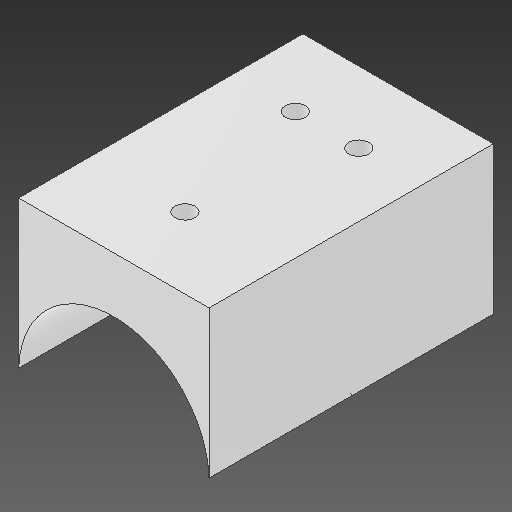
# Autodesk Inventor part: TopMotorMountSandwich3DPrint
Saved by Autodesk Inventor 2021 (Build 250183000, 183)
## iProperties
Created: 2021-02-22
Part Number: TopMotorMountSandwich3DPrint
Material: PC/ABS Plastic
Document SubType Name: Modeling
Designer: Esketitttttt
Density: 0.357273 g/cm^3
Appearance: Smooth - White
Mass: 0.946273 g
Surface Area: 18.8955 cm^2
Volume: 2.6486 cm^3
Author: Esketitttttt
Autodesk Inventor part; units mm, degrees
ref_plane "YZ Plane" through (0, 0, 0) normal (1, 0, 0) x (0, 1, 0)
ref_plane "XZ Plane" through (0, 0, 0) normal (0, 1, 0) x (-1, 0, 0)
ref_plane "XY Plane" through (0, 0, 0) normal (0, 0, 1) x (1, 0, 0)
sketch "Sketch1" plane through (0, 0, 0) normal (0, 0, 1) x (1, 0, 0)
  circle A0 centre (0, 0) radius 8.04
  line L0 (6, 4.8139) -> (6, -4.8139)
  arc A1 (6, 4.8139) -> (5.9407, 4.977) centre (5.746, 4.8139) ccw
  arc A2 (5.9407, 4.977) -> (-5.9407, 4.977) centre (0, 0) ccw
  arc A3 (-5.9407, 4.977) -> (-6, 4.8139) centre (-5.746, 4.8139) ccw
  line L1 (-6, -4.8139) -> (-6, 4.8139)
  arc A4 (-6, -4.8139) -> (-5.9407, -4.977) centre (-5.746, -4.8139) ccw
  arc A5 (-5.9407, -4.977) -> (5.9407, -4.977) centre (0, 0) ccw
  arc A6 (5.9407, -4.977) -> (6, -4.8139) centre (5.746, -4.8139) ccw
  line L2 (0, 8.04) -> (-12.7, 8.04)
  line L3 (0, 8.04) -> (12.7, 8.04) construction
  line L4 (-12.7, 8.04) -> (12.7, 8.04)
  line L5 (12.7, 8.04) -> (12.7, -8.04)
  line L6 (12.7, -8.04) -> (-12.7, -8.04)
  line L7 (-12.7, -8.04) -> (-12.7, 8.04)
  line L8 (0, -8.04) -> (0, 8.04)
  line L9 (0, 8.04) -> (0.254, 8.04)
  line L10 (0.254, 8.04) -> (0.254, -8.04)
  line L11 (0.254, -8.04) -> (0, -8.04)
  line L12 (0, -8.04) -> (0, 8.04)
  point P0 (0, -8.04)
  point P1 (0, -7.75)
  point P2 (0, 7.75)
  point P3 (0.254, 8.036)
  point P4 (0.254, -8.036)
  point P5 (0.254, -7.7458)
  point P6 (0.254, 7.7458)
  dimension "d0" = 12.7
  dimension "d2" = 25.4
  dimension "d7" = 0.254
  constraints: 26 end point, 12 point on circle, 6 centre point, 5 horizontal, 4 parallel, 2 perpendicular, 1 collinear, 1 midpoint, 1 point on line, 3 other
  measures "d0" distance of L2.start L2.end
  measures "d2" distance of L5.end L6.end
  measures "d7" distance of L10.end L11.end
extrude "Extrusion1" add sketch "Sketch1" along normal blind 12 contours L10 L4 L5 L6 A0
extrude "Extrusion2" add sketch "Sketch1" against normal blind 12 contours L10 L4 L5 L6 A0 | A0 L10 A5 A6 L0 A1 A2
sketch "Sketch2" plane through (12.7, -8.04, 12) normal (1, 0, 0) x (0, 0, -1)
  line L0 (12, 12.8539) -> (12, 3.2261) projected
  line L1 (24, 16.08) -> (24, 0) construction
  line L2 (24, 0) -> (0, 0) projected
  line L3 (24, 16.08) -> (12, 16.08)
  line L4 (12, 16.08) -> (12, 0)
  line L5 (12, 0) -> (24, 0)
  line L6 (24, 0) -> (24, 16.08) construction
  line L7 (24, 16.08) -> (0, 16.08) projected
  line L8 (12, 16.08) -> (24, 0) construction
  line L9 (12, 16.08) -> (16, 10.72) construction
  line L10 (16, 10.72) -> (20, 5.36) construction
  line L11 (12, 16.076) -> (0, 16.076) projected
  line L12 (12, 0) -> (0, 16.076)
  line L13 (24, 16.08) -> (18, 16.08)
  line L14 (18, 16.08) -> (18, 10.72)
  line L15 (18, 10.72) -> (24, 10.72)
  line L16 (24, 10.72) -> (24, 16.08)
  line L17 (24, 10.72) -> (18, 10.72)
  line L18 (18, 10.72) -> (18, 5.36)
  line L19 (18, 5.36) -> (24, 5.36)
  line L20 (24, 5.36) -> (24, 10.72)
  line L21 (0, 0) -> (0, 16.08) projected
  point P0 (12, 8.04)
  point P1 (6, 8.038)
  dimension "d18" = 20.0641
  dimension "d19" = 6.688
  dimension "d20" = 6.688
  dimension "d21" = 12
  dimension "d22" = 16.08
  dimension "d23" = 6
  dimension "d24" = 5.36
  dimension "d25" = 6
  dimension "d26" = 5.36
  dimension "d27" = 12
  constraints: 32 end point, 6 parallel, 5 coincident, 3 horizontal, 3 perpendicular, 2 midpoint, 2 point on line
  measures "d18" distance of L3.end L5.end
  measures "d19" distance of L3.end L9.end
  measures "d20" distance of L9.end L10.end
  measures "d21" distance of L1.start L3.end
  measures "d22" distance of L1.start L1.end
  measures "d23" distance of L15.end L14.end
  measures "d24" distance of L14.end L13.end
  measures "d25" distance of L19.end L18.end
  measures "d26" distance of L18.end L17.end
  measures "d27" distance between parallel lines of L21 L0
hole "Hole1" at (12.7, -0.002, 6) at (12.7, 2.68, -6) at (12.7, -2.68, -6) direction (-1, 0, 0) diameter 1.7018 depth 9.525 tip angle 118
equation "\"d19\" = 0.333333 * d18"
equation "\"d20\" = 0.333333 * d18"
equation "\"d23\" = 0.5 * d21"
equation "\"d24\" = 0.333333 * d22"
equation "\"d25\" = d23"
equation "\"d26\" = d24"
body "Solid1"
